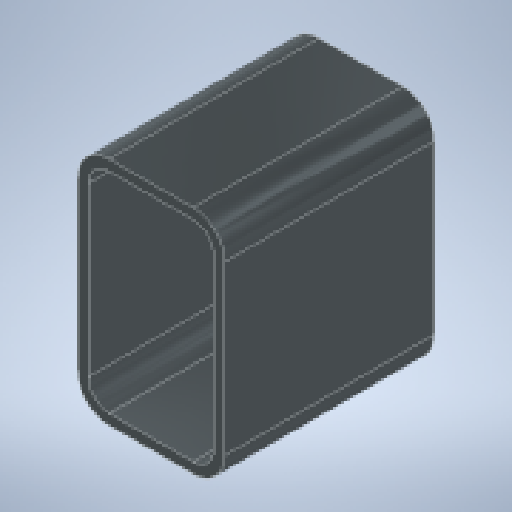
# Autodesk Inventor part: class1
Saved by Autodesk Inventor 2024.2 (Build 282272000, 272)
## iProperties
Created: 2024-07-24
Part Number: class1
Material: Iron, Ductile
Document SubType Name: Modeling
Designer: eamon
Density: 7.15 g/cm^3
Appearance: Iron Gray
Author: eamon
Autodesk Inventor part; units mm, degrees
ref_plane "YZ Plane" through (0, 0, 0) normal (1, 0, 0) x (0, 1, 0)
ref_plane "XZ Plane" through (0, 0, 0) normal (0, 1, 0) x (-1, 0, 0)
ref_plane "XY Plane" through (0, 0, 0) normal (0, 0, 1) x (1, 0, 0)
sketch "Sketch1" plane through (0, 0, 0) normal (0, 0, 1) x (1, 0, 0)
  line L0 (-25.4, 63.5) -> (25.4, 63.5)
  line L1 (38.1, 50.8) -> (38.1, -50.8)
  line L2 (25.4, -63.5) -> (-25.4, -63.5)
  line L3 (-38.1, -50.8) -> (-38.1, 50.8)
  line L4 (-38.1, 63.5) -> (38.1, -63.5) construction
  line L5 (38.1, 63.5) -> (-38.1, -63.5) construction
  arc A0 (-25.4, 63.5) -> (-38.1, 50.8) centre (-25.4, 50.8) ccw
  arc A1 (38.1, 50.8) -> (25.4, 63.5) centre (25.4, 50.8) ccw
  arc A2 (25.4, -63.5) -> (38.1, -50.8) centre (25.4, -50.8) ccw
  arc A3 (-38.1, -50.8) -> (-25.4, -63.5) centre (-25.4, -50.8) ccw
  line L6 (25.4, 69.85) -> (-25.4, 69.85)
  arc A4 (-25.4, 69.85) -> (-44.45, 50.8) centre (-25.4, 50.8) ccw
  line L7 (-44.45, 50.8) -> (-44.45, -50.8)
  arc A5 (-44.45, -50.8) -> (-25.4, -69.85) centre (-25.4, -50.8) ccw
  line L8 (-25.4, -69.85) -> (25.4, -69.85)
  arc A6 (25.4, -69.85) -> (44.45, -50.8) centre (25.4, -50.8) ccw
  line L9 (44.45, -50.8) -> (44.45, 50.8)
  arc A7 (44.45, 50.8) -> (25.4, 69.85) centre (25.4, 50.8) ccw
  point P0 (0, 0)
  dimension "d0" = 127
  dimension "d1" = 76.2
  dimension "d2" = 12.7
  dimension "d3" = 6.35
  constraints: 20 end point, 16 point on circle, 8 centre point, 8 point on line, 8 tangent, 4 parallel, 3 equal radius, 2 midpoint, 2 perpendicular, 1 horizontal, 7 other
  measures "d0" distance of L5.start L4.end
  measures "d1" distance of L4.end L5.end
  measures "d2" radius of A0
  measures "d3" distance between parallel lines of L0 L6
extrude "Extrusion1" add sketch "Sketch1" against normal blind 127
body "Solid1"
